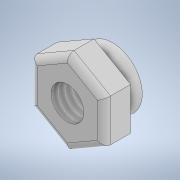
# Autodesk Inventor part: BOB-M3-2-3W
Saved by Autodesk Inventor 2020 (Build 240168000, 168)
## iProperties
Created: 2020-06-27
Part Number: BOB-M3-2-3W
Material: 一般
Document SubType Name: Modeling
Designer: haya
Density: 1 g/cm^3
Appearance: 既定
Author: haya
Autodesk Inventor part; units mm, degrees
ref_plane "YZ Plane" through (0, 0, 0) normal (1, 0, 0) x (0, 1, 0)
ref_plane "XZ Plane" through (0, 0, 0) normal (0, 1, 0) x (-1, 0, 0)
ref_plane "XY Plane" through (0, 0, 0) normal (0, 0, 1) x (1, 0, 0)
sketch "スケッチ1" plane through (0, 0, 0) normal (0, 0, 1) x (1, 0, 0)
  line L0 (0, -3.1754) -> (-2.75, -1.5877)
  line L1 (-2.75, -1.5877) -> (-2.75, 1.5877)
  line L2 (-2.75, 1.5877) -> (0, 3.1754)
  line L3 (0, 3.1754) -> (2.75, 1.5877)
  line L4 (2.75, 1.5877) -> (2.75, -1.5877)
  line L5 (2.75, -1.5877) -> (0, -3.1754)
  point P0 (0, 0)
  point P1 (0, 0)
  dimension "d0" = 5.5
  constraints: 12 end point, 1 coincident, 13 other
  measures "d0" distance between parallel lines of L4 L1
extrude "押し出し1" add sketch "スケッチ1" along normal blind 2
sketch "スケッチ2" plane through (0, 0, 0) normal (0, 0, -1) x (-1, 0, 0)
  circle A0 centre (0, 0) radius 2.225
  dimension "d3" = 4.45
  constraints: 1 centre point, 1 coincident
  measures "d3" diameter of A0
extrude "押し出し2" add sketch "スケッチ2" along normal blind 1.4
sketch "スケッチ3" plane through (0, 0, -1.4) normal (0, 0, -1) x (-1, 0, 0)
  point P0 (0, 0)
hole "穴1" at (0, 0, -1.4) direction (0, 0, 1) diameter 2.459 end through all thread size "M3x0.5" class "6H" standard "ISO Metric profile"
fillet "フィレット1" radius 0.5 6 edges at (1.375, 2.3816, 2) (2.75, 0, 2) (1.375, -2.3816, 2) (-1.375, -2.3816, 2) (-2.75, 0, 2) (-1.375, 2.3816, 2)
